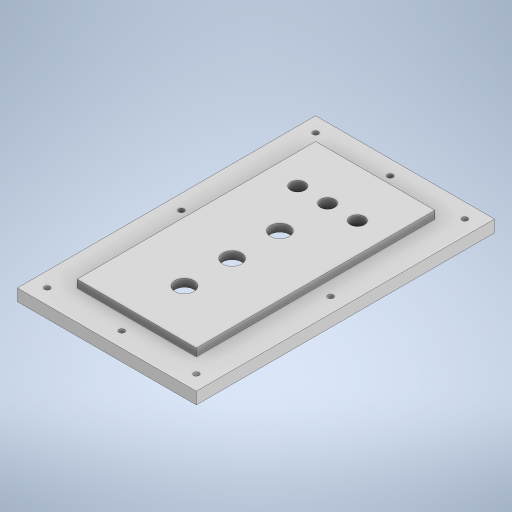
# Autodesk Inventor part: Faceplate
Saved by Autodesk Inventor 2024 (Build 280153020, 153B)
## iProperties
Created: 2023-07-16
Part Number: Faceplate
Material: Generic
Document SubType Name: Modeling
Designer: torban
Density: 1 g/cm^3
Appearance: Default
Author: torban
Autodesk Inventor part; units mm, degrees
ref_plane "YZ Plane" through (0, 0, 0) normal (1, 0, 0) x (0, 1, 0)
ref_plane "XZ Plane" through (0, 0, 0) normal (0, 1, 0) x (-1, 0, 0)
ref_plane "XY Plane" through (0, 0, 0) normal (0, 0, 1) x (1, 0, 0)
sketch "Sketch1" plane through (0, 0, 0) normal (0, 1, 0) x (-1, 0, 0)
  line L0 (0, 0) -> (100, 0)
  line L1 (100, 0) -> (100, -200)
  line L2 (100, -200) -> (0, -200)
  line L3 (0, -200) -> (0, 0)
  dimension "d0" = 200
  dimension "d1" = 100
  constraints: 8 end point, 2 parallel, 1 horizontal, 1 perpendicular
  measures "d0" distance of L0.end L1.end
  measures "d1" distance of L1.end L2.end
extrude "Extrusion1" add sketch "Sketch1" along normal blind 6.35
sketch "Sketch2" plane through (0, 0, 0) normal (0, -1, 0) x (1, 0, 0)
  line L0 (0, 0) -> (0, -200) projected
  line L1 (0, -200) -> (-100, -200) projected
  line L2 (-100, -200) -> (-100, 0) projected
  line L3 (-100, 0) -> (0, 0) projected
  line L4 (25, 25) -> (25, -225)
  line L5 (25, -225) -> (-125, -225)
  line L6 (-125, -225) -> (-125, 25)
  line L7 (-125, 25) -> (25, 25)
  dimension "d4" = 25
  constraints: 8 end point, 3 other
  measures "d4" distance between parallel lines of L3 L7
extrude "Extrusion2" add sketch "Sketch2" along normal blind 10 contours L0 L1 L2 L3 | L4 L5 L6 L7
sketch "Sketch3" plane through (0, 0, 0) normal (0, 1, 0) x (1, 0, 0)
  line L0 (-125, -25) -> (-125, 225) projected
  line L1 (-125, 225) -> (25, 225) projected
  line L2 (25, 225) -> (25, -25) projected
  line L3 (25, -25) -> (-125, -25) projected
  line L4 (0, 0) -> (0, 200) projected
  line L5 (0, 200) -> (-100, 200) projected
  line L6 (-100, 200) -> (-100, 0) projected
  line L7 (-100, 0) -> (0, 0) projected
  line L8 (12.5, -12.5) -> (12.5, 212.5)
  line L9 (12.5, 212.5) -> (-112.5, 212.5)
  line L10 (-112.5, 212.5) -> (-112.5, -12.5)
  line L11 (-112.5, -12.5) -> (12.5, -12.5)
  point P0 (12.5, 100)
  point P1 (-112.5, 100)
  point P2 (-50, 212.5)
  point P3 (-50, -12.5)
  dimension "d7" = 12.5
  constraints: 8 end point, 4 coincident, 4 midpoint, 3 other
  measures "d7" distance between parallel lines of L7 L11
hole "Hole1" at (-112.5, 0, 12.5) at (12.5, 0, 12.5) at (-112.5, 0, -212.5) at (12.5, 0, -212.5) at (12.5, 0, -100) at (-112.5, 0, -100) at (-50, 0, -212.5) at (-50, 0, 12.5) direction (0, -1, 0) diameter 4.69 end through all
sketch "Sketch4" plane through (0, 6.35, 0) normal (0, 1, 0) x (1, 0, 0)
  line L0 (-100, 0) -> (0, 0) construction
  line L1 (-75, 0) -> (-75, 200) construction
  line L2 (0, 200) -> (-100, 200) construction
  line L3 (0, 0) -> (0, 200) construction
  line L4 (-100, 200) -> (-100, 0) construction
  line L5 (-50, 0) -> (-50, 200) construction
  line L6 (-100, 40) -> (0, 40) construction
  line L7 (-100, 120) -> (0, 120) construction
  line L8 (-100, 80) -> (0, 80) construction
  line L9 (-25, 0) -> (-25, 200) construction
  line L10 (-100, 160) -> (0, 160) construction
  circle A0 centre (-50, 120) radius 8
  circle A1 centre (-50, 80) radius 8
  circle A2 centre (-50, 40) radius 8
  circle A3 centre (-75, 160) radius 2.6
  circle A4 centre (-50, 160) radius 2.6
  circle A5 centre (-25, 160) radius 2.6
  dimension "d15" = 100
  dimension "d16" = 25
  dimension "d17" = 200
  dimension "d18" = 25
  dimension "d19" = 40
  dimension "d20" = 40
  dimension "d21" = 40
  dimension "d22" = 25
  dimension "d23" = 40
  dimension "d24" = 16
  dimension "d25" = 16
  dimension "d26" = 16
  dimension "d27" = 5.2
  dimension "d28" = 5.2
  dimension "d29" = 5.2
  dimension "d30" = 0
  dimension "d31" = 50
  constraints: 14 end point, 14 point on line, 6 centre point, 6 coincident, 6 midpoint, 5 perpendicular, 1 parallel, 1 vertical
  measures "d15" distance between parallel lines of L3 L4
  measures "d16" distance between parallel lines of L4 L1
  measures "d17" distance between parallel lines of L2 L0
  measures "d18" distance between parallel lines of L1 L5
  measures "d19" distance between parallel lines of L6 L0
  measures "d20" distance between parallel lines of L6 L8
  measures "d21" distance between parallel lines of L7 L8
  measures "d22" distance between parallel lines of L5 L9
  measures "d23" distance between parallel lines of L7 L10
  measures "d24" diameter of A0
  measures "d25" diameter of A1
  measures "d26" diameter of A2
  measures "d27" diameter of A3
  measures "d28" diameter of A4
  measures "d29" diameter of A5
  measures "d30" distance from line of L10.end L3
  measures "d31" distance from line of point (-50, 160) L3
extrude "Extrusion3" cut sketch "Sketch4" against normal through all
sketch "Sketch5" plane through (0, -10, 0) normal (0, -1, 0) x (1, 0, 0)
  circle A0 centre (-50, -40) radius 8 projected
  circle A1 centre (-25, -160) radius 2.6 projected
  circle A2 centre (-50, -80) radius 8 projected
  circle A3 centre (-75, -160) radius 2.6 projected
  circle A4 centre (-50, -160) radius 2.6 projected
  circle A5 centre (-50, -120) radius 8 projected
  line L0 (0, -200) -> (-100, -200) projected
  line L1 (-100, -200) -> (-100, 0) projected
  line L2 (-100, 0) -> (0, 0) projected
  line L3 (0, 0) -> (0, -200) projected
extrude "Extrusion4" cut sketch "Sketch5" against normal blind 9.9
chamfer "Chamfer1" distance 9.9 angle 45 4 edges at (0, -0.1, -100) (-50, -0.1, 0) (-100, -0.1, -100) (-50, -0.1, -200)
sketch "Sketch9" plane through (0, -0.1, 0) normal (0, -1, 0) x (1, 0, 0)
  line L0 (-9.9, -9.9) -> (-90.1, -9.9) projected
  line L1 (-90.1, -9.9) -> (-90.1, -190.1) projected
  line L2 (-90.1, -190.1) -> (-9.9, -190.1) projected
  line L3 (-9.9, -190.1) -> (-9.9, -9.9) projected
  circle A0 centre (-50, -40) radius 8 projected
  circle A1 centre (-25, -160) radius 2.6 projected
  circle A2 centre (-50, -80) radius 8 projected
  circle A3 centre (-75, -160) radius 2.6 projected
  circle A4 centre (-50, -160) radius 2.6 projected
  circle A5 centre (-50, -120) radius 8 projected
  circle A6 centre (-50, 12.5) radius 2.345 projected
  circle A7 centre (-50, -212.5) radius 2.345 projected
  circle A8 centre (-112.5, -100) radius 2.345 projected
  circle A9 centre (12.5, -100) radius 2.345 projected
  circle A10 centre (12.5, -212.5) radius 2.345 projected
  circle A11 centre (-112.5, -212.5) radius 2.345 projected
  circle A12 centre (12.5, 12.5) radius 2.345 projected
  circle A13 centre (-112.5, 12.5) radius 2.345 projected
  line L4 (-125, 25) -> (25, 25) projected
  line L5 (25, 25) -> (25, -225) projected
  line L6 (25, -225) -> (-125, -225) projected
  line L7 (-125, -225) -> (-125, 25) projected
  circle A14 centre (-25, -160) radius 6
  circle A15 centre (-50, -160) radius 6
  circle A16 centre (-75, -160) radius 6
  point P0 (0, 0)
  dimension "d44" = 12
  dimension "d45" = 12
  dimension "d46" = 12
  constraints: 3 centre point, 3 coincident
  measures "d44" diameter of A14
  measures "d45" diameter of A15
  measures "d46" diameter of A16
extrude "Extrusion6" add sketch "Sketch9" along normal blind 5 contours A14 | A15 | A16
chamfer "Chamfer2" distance 5 angle 45 3 edges at (-31, -0.1, -160) (-56, -0.1, -160) (-81, -0.1, -160)
sketch "Sketch10" plane through (0, 6.35, 0) normal (0, 1, 0) x (1, 0, 0)
  circle A0 centre (-50, 160) radius 6 projected
  circle A1 centre (-50, 160) radius 2.6 projected
  circle A2 centre (-75, 160) radius 6 projected
  circle A3 centre (-75, 160) radius 2.6 projected
  circle A4 centre (-25, 160) radius 6 projected
  circle A5 centre (-25, 160) radius 2.6 projected
  point P0 (0, 0)
extrude "Extrusion7" cut sketch "Sketch10" against normal blind 8
equation "\"d16\" = 0.25 * d15"
equation "\"d18\" = d16"
equation "\"d19\" = 0.2 * d17"
equation "\"d20\" = d19"
equation "\"d21\" = d20"
equation "\"d22\" = d18"
equation "\"d23\" = d21"
equation "\"d28\" = d27"
equation "\"d29\" = d27"
body "Solid1"
